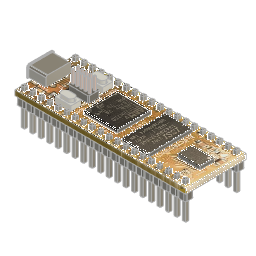
Seed Cover v4 (Autodesk Fusion 360 archive; units mm, degrees)
design "Daisy Board"
Autodesk Fusion 360 part; units mm, degrees
(part 1 of 2)
box "BoxPrimitive1" add length 18.11 width 51.14 height 1.53 placed x (0, -1, 0) y (1, 0, 0) z (0, 0, 1) at (-75.0693, 56.4508, 0) makes body 1
sketch "Sketch3" plane through (0, 0, 1.53) normal (0, 0, 1) x (-1, 0, 0)
  line L0 (75.0693, -38.3408) -> (23.9293, -38.3408)
  line L1 (23.9293, -38.3408) -> (23.9293, -56.4508)
  line L2 (23.9293, -56.4508) -> (75.0693, -56.4508)
  line L3 (75.0693, -56.4508) -> (75.0693, -38.3408)
  line L4 (23.9293, -47.3958) -> (37.4493, -47.3958) construction
  line L5 (37.4493, -56.4508) -> (37.4493, -38.3408) construction
  line L6 (37.4493, -47.3958) -> (45.4493, -47.3958) construction
  line L7 (45.4493, -56.4508) -> (45.4493, -38.3408) construction
  line L8 (45.4493, -47.3958) -> (48.3593, -47.3958) construction
  line L9 (48.3593, -56.4508) -> (48.3593, -38.3408) construction
  line L10 (48.3593, -47.3958) -> (58.3893, -47.3958) construction
  line L11 (58.3893, -56.4508) -> (58.3893, -38.3408) construction
  line L12 (58.3893, -47.3958) -> (60.3893, -47.3958) construction
  line L13 (60.3893, -56.4508) -> (60.3893, -38.3408) construction
  line L14 (60.3893, -47.3958) -> (66.5893, -47.3958) construction
  line L15 (66.5893, -56.4508) -> (66.5893, -38.3408) construction
  line L16 (66.5893, -47.3958) -> (71.0293, -47.3958) construction
  line L17 (71.0293, -56.4508) -> (71.0293, -38.3408) construction
  line L18 (71.0293, -47.3958) -> (76.5893, -47.3958) construction
  line L19 (76.5893, -56.4508) -> (76.5893, -38.3408) construction
  line L20 (23.9293, -47.3958) -> (26.5293, -47.3958) construction
  line L21 (26.5293, -56.4508) -> (26.5293, -38.3408) construction
  line L22 (26.5293, -47.3958) -> (33.1493, -47.3958) construction
  line L23 (33.1493, -56.4508) -> (33.1493, -38.3408) construction
  line L24 (33.1493, -47.3958) -> (33.1493, -49.5458) construction
  line L25 (33.1493, -47.3958) -> (33.1493, -45.2458) construction
  line L26 (33.1493, -49.5458) -> (26.5293, -49.5458)
  line L27 (26.5293, -49.5458) -> (26.5293, -45.2458)
  line L28 (26.5293, -45.2458) -> (33.1493, -45.2458)
  line L29 (33.1493, -45.2458) -> (33.1493, -49.5458)
  line L30 (37.4493, -47.3958) -> (37.4493, -53.8958) construction
  line L31 (37.4493, -47.3958) -> (37.4493, -40.8958) construction
  line L32 (37.4493, -53.8958) -> (45.4493, -53.8958)
  line L33 (45.4493, -53.8958) -> (45.4493, -40.8958)
  line L34 (45.4493, -40.8958) -> (37.4493, -40.8958)
  line L35 (37.4493, -40.8958) -> (37.4493, -53.8958)
  line L36 (48.3593, -47.3958) -> (48.3593, -52.4158) construction
  line L37 (48.3593, -47.3958) -> (48.3593, -42.3758) construction
  line L38 (48.3593, -52.4158) -> (58.3893, -52.4158)
  line L39 (58.3893, -52.4158) -> (58.3893, -42.3758)
  line L40 (58.3893, -42.3758) -> (48.3593, -42.3758)
  line L41 (48.3593, -42.3758) -> (48.3593, -52.4158)
  line L42 (60.3893, -47.3958) -> (60.3893, -49.0758) construction
  line L43 (60.3893, -47.3958) -> (60.3893, -45.7158) construction
  line L44 (60.3893, -45.7158) -> (66.5893, -45.7158)
  line L45 (66.5893, -45.7158) -> (66.5893, -49.0758)
  line L46 (66.5893, -49.0758) -> (60.3893, -49.0758)
  line L47 (60.3893, -49.0758) -> (60.3893, -45.7158)
  line L48 (71.0293, -47.3958) -> (71.0293, -51.1708) construction
  line L49 (71.0293, -47.3958) -> (71.0293, -43.6208) construction
  line L50 (71.0293, -51.1708) -> (76.5893, -51.1708)
  line L51 (76.5893, -51.1708) -> (76.5893, -43.6208)
  line L52 (76.5893, -43.6208) -> (71.0293, -43.6208)
  line L53 (71.0293, -43.6208) -> (71.0293, -51.1708)
  line L54 (66.5893, -49.0758) -> (66.5893, -50.5758) construction
  line L55 (66.5893, -45.7158) -> (66.5893, -44.2158) construction
  line L56 (65.9033, -38.3408) -> (65.9033, -56.4508) construction
  line L57 (61.0338, -38.3408) -> (61.0338, -56.4508) construction
  line L58 (65.9033, -50.5758) -> (61.0338, -50.5758)
  line L59 (61.0338, -50.5758) -> (61.0338, -53.7158)
  line L60 (61.0338, -53.7158) -> (65.9033, -53.7158)
  line L61 (65.9033, -53.7158) -> (65.9033, -50.5758)
  line L62 (65.9033, -44.2158) -> (61.0338, -44.2158)
  line L63 (61.0338, -44.2158) -> (61.0338, -41.0758)
  line L64 (61.0338, -41.0758) -> (65.9033, -41.0758)
  line L65 (65.9033, -41.0758) -> (65.9033, -44.2158)
  line L66 (64.4033, -51.0758) -> (62.5338, -51.0758)
  line L67 (61.5338, -52.0758) -> (61.5338, -52.2158)
  line L68 (62.5338, -53.2158) -> (64.4033, -53.2158)
  line L69 (65.4033, -52.2158) -> (65.4033, -52.0758)
  line L70 (62.5338, -41.5758) -> (64.4033, -41.5758)
  line L71 (65.4033, -42.5758) -> (65.4033, -42.7158)
  line L72 (64.4033, -43.7158) -> (62.5338, -43.7158)
  line L73 (61.5338, -42.7158) -> (61.5338, -42.5758)
  arc A0 (64.4033, -53.2158) -> (65.4033, -52.2158) centre (64.4033, -52.2158) ccw
  arc A1 (61.5338, -52.2158) -> (62.5338, -53.2158) centre (62.5338, -52.2158) ccw
  arc A2 (62.5338, -51.0758) -> (61.5338, -52.0758) centre (62.5338, -52.0758) ccw
  arc A3 (65.4033, -52.0758) -> (64.4033, -51.0758) centre (64.4033, -52.0758) ccw
  arc A4 (64.4033, -43.7158) -> (65.4033, -42.7158) centre (64.4033, -42.7158) ccw
  arc A5 (61.5338, -42.7158) -> (62.5338, -43.7158) centre (62.5338, -42.7158) ccw
  arc A6 (62.5338, -41.5758) -> (61.5338, -42.5758) centre (62.5338, -42.5758) ccw
  arc A7 (65.4033, -42.5758) -> (64.4033, -41.5758) centre (64.4033, -42.5758) ccw
  dimension "d7" = 13.52
  dimension "d8" = 8
  dimension "d9" = 2.91
  dimension "d10" = 10.03
  dimension "d11" = 2
  dimension "d12" = 6.2
  dimension "d13" = 4.44
  dimension "d14" = 5.56
  dimension "d15" = 2.6
  dimension "d16" = 6.62
  dimension "d17" = 2.15
  dimension "d18" = 2.15
  dimension "d19" = 6.5
  dimension "d20" = 6.5
  dimension "d21" = 5.02
  dimension "d22" = 5.02
  dimension "d23" = 1.68
  dimension "d24" = 1.68
  dimension "d25" = 3.775
  dimension "d26" = 3.775
  dimension "d49" = 1.5
  dimension "d50" = 1.5
  dimension "d51" = 3.14
  dimension "d52" = 3.14
  dimension "d55" = 1
  constraint midpoint L1 L4.start
  constraint perpendicular L1 L4
  constraint coincident L2 L5.start
  constraint coincident L0 L5.end
  constraint perpendicular L0 L5
  constraint perpendicular L5 L6
  constraint coincident L2 L7.start
  constraint coincident L0 L7.end
  constraint perpendicular L0 L7
  constraint perpendicular L7 L8
  constraint coincident L2 L9.start
  constraint coincident L0 L9.end
  constraint perpendicular L0 L9
  constraint perpendicular L9 L10
  constraint coincident L2 L11.start
  constraint coincident L0 L11.end
  constraint perpendicular L0 L11
  constraint perpendicular L11 L12
  constraint coincident L2 L13.start
  constraint coincident L0 L13.end
  constraint perpendicular L0 L13
  constraint perpendicular L13 L14
  constraint coincident L2 L15.start
  constraint coincident L0 L15.end
  constraint perpendicular L0 L15
  constraint perpendicular L15 L16
  constraint coincident L2 L17.start
  constraint coincident L0 L17.end
  constraint perpendicular L0 L17
  constraint perpendicular L3 L18
  constraint perpendicular L0 L19
  constraint perpendicular L1 L20
  constraint coincident L2 L21.start
  constraint coincident L0 L21.end
  constraint perpendicular L0 L21
  constraint perpendicular L21 L22
  constraint coincident L2 L23.start
  constraint coincident L0 L23.end
  constraint perpendicular L0 L23
  constraint perpendicular L4 L24
  constraint perpendicular L4 L25
  constraint horizontal L26
  constraint vertical L27
  constraint horizontal L28
  constraint vertical L29
  constraint coincident L21 L27.end
  constraint perpendicular L6 L30
  constraint perpendicular L6 L31
  constraint horizontal L32
  constraint vertical L33
  constraint horizontal L34
  constraint vertical L35
  constraint coincident L7 L33.end
  constraint perpendicular L10 L36
  constraint perpendicular L10 L37
  constraint horizontal L38
  constraint vertical L39
  constraint horizontal L40
  constraint vertical L41
  constraint coincident L11 L39.end
  constraint perpendicular L14 L42
  constraint perpendicular L14 L43
  constraint horizontal L44
  constraint vertical L45
  constraint horizontal L46
  constraint vertical L47
  constraint coincident L15 L45.end
  constraint perpendicular L18 L48
  constraint perpendicular L16 L49
  constraint horizontal L50
  constraint vertical L51
  constraint horizontal L52
  constraint vertical L53
  constraint coincident L19 L51.end
  constraint perpendicular L46 L54
  constraint perpendicular L44 L55
  constraint coincident L0 L56.start
  constraint coincident L2 L56.end
  constraint perpendicular L2 L56
  constraint coincident L0 L57.start
  constraint perpendicular L46 L57
  constraint horizontal L58
  constraint vertical L59
  constraint horizontal L60
  constraint vertical L61
  constraint coincident L56 L58.start
  constraint horizontal L62
  constraint vertical L63
  constraint horizontal L64
  constraint vertical L65
  constraint coincident L56 L62.start
  constraint parallel L58 L66
  constraint parallel L59 L67
  constraint parallel L60 L68
  constraint parallel L61 L69
  constraint tangent L68 A0
  constraint tangent L69 A0
  constraint tangent L67 A1
  constraint tangent L68 A1
  constraint equal A0 A1
  constraint tangent L66 A2
  constraint tangent L67 A2
  constraint equal A0 A2
  constraint tangent L66 A3
  constraint tangent L69 A3
  constraint equal A0 A3
  constraint parallel L64 L70
  constraint parallel L65 L71
  constraint parallel L62 L72
  constraint parallel L63 L73
  constraint tangent L71 A4
  constraint tangent L72 A4
  constraint equal A0 A4
  constraint tangent L72 A5
  constraint tangent L73 A5
  constraint equal A0 A5
  constraint tangent L70 A6
  constraint tangent L73 A6
  constraint equal A0 A6
  constraint tangent L70 A7
  constraint tangent L71 A7
  constraint equal A0 A7
  measures "d7" distance of L4.start L4.end
  measures "d8" distance of L4.end L6.end
  measures "d9" distance of L6.end L8.end
  measures "d10" distance of L8.end L10.end
  measures "d11" distance of L10.end L12.end
  measures "d12" distance of L12.end L14.end
  measures "d13" distance of L14.end L16.end
  measures "d14" distance of L16.end L18.end
  measures "d15" distance of L4.start L20.end
  measures "d16" distance of L20.end L22.end
  measures "d17" distance of L22.end L24.end
  measures "d18" distance of L22.end L25.end
  measures "d19" distance of L4.end L30.end
  measures "d20" distance of L4.end L31.end
  measures "d21" distance of L8.end L36.end
  measures "d22" distance of L8.end L37.end
  measures "d23" distance of L12.end L42.end
  measures "d24" distance of L12.end L43.end
  measures "d25" distance of L16.end L48.end
  measures "d26" distance of L16.end L49.end
  measures "d49" distance of L45.end L54.end
  measures "d50" distance of L44.end L55.end
  measures "d51" distance of L58.start L60.end
  measures "d52" distance of L62.start L64.end
  measures "d55" radius of A0
extrude "Extrude1" add sketch "Sketch3" along normal blind 1 separate body contours L26 L27 L28 L29 makes body 2
extrude "Extrude2" add sketch "Sketch3" along normal blind 1 separate body contours L32 L33 L34 L35 makes body 3
extrude "Extrude3" add sketch "Sketch3" along normal blind 1 separate body contours L38 L39 L40 L41 makes body 4
extrude "Extrude4" add sketch "Sketch3" along normal blind 2 separate body contours L44 L45 L46 L47 makes body 5
extrude "Extrude5" add sketch "Sketch3" along normal blind 3 separate body contours L3 L50 L51 L52 | L3 L50 L52 L53 makes body 6
fillet "Fillet1" radius 0.5 2 edges at (-73.8093, 51.1708, 4.53) (-73.8093, 43.6208, 4.53) on bodies 6
fillet "Fillet2" radius 0.25 tangency weight 0.80688 4 edges at (-66.5893, 45.7158, 2.53) (-66.5893, 49.0758, 2.53) (-60.3893, 49.0758, 2.53) (-60.3893, 45.7158, 2.53) on bodies 5
sketch "Sketch4" plane through (0, 0, 3.53) normal (0, 0, 1) x (-1, 0, 0)
  spline S0 degree 3 poles (60.3893, -45.9658) (60.3893, -45.9427) (60.3942, -45.9181) (60.4159, -45.8622) (60.435, -45.8319) (60.4862, -45.776) (60.5184, -45.7522) (60.5671, -45.7296) (60.5826, -45.7241) (60.6118, -45.7175) (60.6256, -45.7158) (60.6393, -45.7158) knots 0 0 0 0 0.006926 0.006926 0.015648 0.015648 0.025212 0.025212 0.029372 0.029372 0.032888 0.032888 0.032888 0.032888
  line L0 (60.3893, -45.9658) -> (60.3893, -48.8258)
  spline S1 degree 3 poles (60.6393, -49.0758) (60.6162, -49.0758) (60.5917, -49.0709) (60.5358, -49.0492) (60.5055, -49.03) (60.4495, -48.9788) (60.4257, -48.9467) (60.4032, -48.898) (60.3977, -48.8825) (60.391, -48.8532) (60.3893, -48.8395) (60.3893, -48.8258) knots 0 0 0 0 0.006926 0.006926 0.015648 0.015648 0.025212 0.025212 0.029372 0.029372 0.032888 0.032888 0.032888 0.032888
  line L1 (60.6393, -49.0758) -> (66.3393, -49.0758)
  spline S2 degree 3 poles (66.5893, -48.8258) (66.5893, -48.8488) (66.5844, -48.8734) (66.5627, -48.9293) (66.5436, -48.9596) (66.4924, -49.0156) (66.4602, -49.0394) (66.4115, -49.0619) (66.396, -49.0674) (66.3668, -49.074) (66.353, -49.0758) (66.3393, -49.0758) knots 0 0 0 0 0.006926 0.006926 0.015648 0.015648 0.025212 0.025212 0.029372 0.029372 0.032888 0.032888 0.032888 0.032888
  line L2 (66.5893, -48.8258) -> (66.5893, -45.9658)
  spline S3 degree 3 poles (66.3393, -45.7158) (66.3624, -45.7158) (66.387, -45.7207) (66.4429, -45.7423) (66.4732, -45.7615) (66.5291, -45.8127) (66.5529, -45.8448) (66.5754, -45.8936) (66.5809, -45.9091) (66.5876, -45.9383) (66.5893, -45.952) (66.5893, -45.9658) knots 0 0 0 0 0.006926 0.006926 0.015648 0.015648 0.025212 0.025212 0.029372 0.029372 0.032888 0.032888 0.032888 0.032888
  line L3 (66.3393, -45.7158) -> (60.6393, -45.7158)
  line L4 (65.7564, -47.944) -> (66.2564, -47.944)
  line L5 (66.2564, -47.944) -> (66.2564, -48.444)
  line L6 (66.2564, -48.444) -> (65.7564, -48.444)
  line L7 (65.7564, -48.444) -> (65.7564, -47.944)
  line L8 (65.7564, -47.944) -> (66.2564, -48.444) construction
  line L9 (66.2564, -47.944) -> (65.7564, -48.444) construction
  line L10 (65.0064, -48.444) -> (64.5064, -48.444)
  line L11 (64.5064, -47.944) -> (65.0064, -47.944)
  line L12 (64.5064, -48.444) -> (64.5064, -47.944)
  line L13 (65.0064, -47.944) -> (65.0064, -48.444)
  line L14 (63.7564, -48.444) -> (63.2564, -48.444)
  line L15 (63.2564, -47.944) -> (63.7564, -47.944)
  line L16 (63.2564, -48.444) -> (63.2564, -47.944)
  line L17 (63.7564, -47.944) -> (63.7564, -48.444)
  line L18 (62.5064, -48.444) -> (62.0064, -48.444)
  line L19 (62.0064, -47.944) -> (62.5064, -47.944)
  line L20 (62.0064, -48.444) -> (62.0064, -47.944)
  line L21 (62.5064, -47.944) -> (62.5064, -48.444)
  line L22 (61.2564, -48.444) -> (60.7564, -48.444)
  line L23 (60.7564, -47.944) -> (61.2564, -47.944)
  line L24 (60.7564, -48.444) -> (60.7564, -47.944)
  line L25 (61.2564, -47.944) -> (61.2564, -48.444)
  line L26 (66.2564, -46.944) -> (65.7564, -46.944)
  line L27 (65.7564, -46.444) -> (66.2564, -46.444)
  line L28 (65.7564, -46.944) -> (65.7564, -46.444)
  line L29 (66.2564, -46.444) -> (66.2564, -46.944)
  line L30 (65.0064, -46.944) -> (64.5064, -46.944)
  line L31 (64.5064, -46.444) -> (65.0064, -46.444)
  line L32 (64.5064, -46.944) -> (64.5064, -46.444)
  line L33 (65.0064, -46.444) -> (65.0064, -46.944)
  line L34 (63.7564, -46.944) -> (63.2564, -46.944)
  line L35 (63.2564, -46.444) -> (63.7564, -46.444)
  line L36 (63.2564, -46.944) -> (63.2564, -46.444)
  line L37 (63.7564, -46.444) -> (63.7564, -46.944)
  line L38 (62.5064, -46.944) -> (62.0064, -46.944)
  line L39 (62.0064, -46.444) -> (62.5064, -46.444)
  line L40 (62.0064, -46.944) -> (62.0064, -46.444)
  line L41 (62.5064, -46.444) -> (62.5064, -46.944)
  line L42 (61.2564, -46.944) -> (60.7564, -46.944)
  line L43 (60.7564, -46.444) -> (61.2564, -46.444)
  line L44 (60.7564, -46.944) -> (60.7564, -46.444)
  line L45 (61.2564, -46.444) -> (61.2564, -46.944)
  point P0 (66.0064, -48.194)
  dimension "d41" = 0.5
  dimension "d42" = 0.5
  dimension "d45" = -5
  dimension "d46" = 1.5
  constraint horizontal L4
  constraint perpendicular L4 L5
  constraint parallel L4 L6
  constraint parallel L5 L7
  constraint coincident L8 P0
  constraint coincident L9 P0
  measures "d41" distance of L5.end L6.end
  measures "d42" distance of L4.end L5.end
extrude "Extrude6" add sketch "Sketch4" along normal blind 4 separate body contours L4 L5 L6 L7 | L10 L11 L12 L13 | L14 L15 L16 L17 | L18 L19 L20 L21 | L22 L23 L24 L25 | L26 L27 L28 L29 | L30 L31 L32 L33 | L34 L35 L36 L37 | L38 L39 L40 L41 | L42 L43 L44 L45 makes body 7 at (-63.5898, 46.944, 4.8633) makes body 8 at (-62.3398, 48.444, 4.8633) makes body 9 at (-64.5064, 48.2774, 4.8633) makes body 10 at (-61.0898, 48.444, 4.8633) makes body 11 at (-64.5064, 46.7774, 4.8633) makes body 12 at (-62.3398, 46.944, 4.8633) makes body 13 at (-63.5898, 48.444, 4.8633) makes body 14 at (-66.2564, 48.1107, 4.8633) makes body 15 at (-61.0898, 46.944, 4.8633) makes body 16 at (-65.7564, 46.7774, 4.8633)
extrude "Extrude7" add sketch "Sketch3" along normal blind 1.5 separate body contours L58 L59 L60 L61 | L62 L63 L64 L65 makes body 17 at (-63.7801, 44.0491, 1.53) makes body 18 at (-63.157, 53.5491, 1.53)
extrude "Extrude8" add sketch "Sketch3" along normal blind 2.5 separate body contours L66 L67 L68 L69 A0 A1 A2 A3 | L70 L71 L72 L73 A4 A5 A6 A7 makes body 19 at (-63.7801, 52.5024, 1.53) makes body 20 at (-63.157, 43.0024, 1.53)
shell "Shell1" thickness 0.3 removed faces 1 at (-76.5893, 48.4874, 2.53) on bodies 6
sketch "Sketch5" plane through (0, 0, 0) normal (0, 0, -1) x (1, 0, 0)
  line L0 (-23.9293, -38.3408) -> (-75.0693, -38.3408)
  line L1 (-75.0693, -38.3408) -> (-75.0693, -56.4508)
  line L2 (-75.0693, -56.4508) -> (-23.9293, -56.4508)
  line L3 (-23.9293, -56.4508) -> (-23.9293, -38.3408)
  line L4 (-74.3757, -41.0103) -> (-72.8757, -41.0103)
  line L5 (-72.3757, -40.5103) -> (-72.3757, -39.0103)
  line L6 (-72.8757, -38.5103) -> (-74.3757, -38.5103)
  line L7 (-74.8757, -39.0103) -> (-74.8757, -40.5103)
  line L8 (-74.1023, -40.2369) -> (-73.1491, -40.2369)
  line L9 (-73.1491, -40.2369) -> (-73.1491, -39.2838)
  line L10 (-73.1491, -39.2838) -> (-74.1023, -39.2838)
  line L11 (-74.1023, -39.2838) -> (-74.1023, -40.2369)
  arc A0 (-74.3757, -38.5103) -> (-74.8757, -39.0103) centre (-74.3757, -39.0103) ccw
  arc A1 (-72.3757, -39.0103) -> (-72.8757, -38.5103) centre (-72.8757, -39.0103) ccw
  arc A2 (-72.8757, -41.0103) -> (-72.3757, -40.5103) centre (-72.8757, -40.5103) ccw
  arc A3 (-74.8757, -40.5103) -> (-74.3757, -41.0103) centre (-74.3757, -40.5103) ccw
  arc A4 (-69.8362, -39.0103) -> (-70.3362, -38.5103) centre (-70.3362, -39.0103) ccw
  line L12 (-70.3362, -38.5103) -> (-71.8362, -38.5103)
  line L13 (-72.3362, -39.0103) -> (-72.3362, -40.5103)
  arc A5 (-71.8362, -38.5103) -> (-72.3362, -39.0103) centre (-71.8362, -39.0103) ccw
  line L14 (-71.5628, -39.2838) -> (-71.5628, -40.2369)
  arc A6 (-72.3362, -40.5103) -> (-71.8362, -41.0103) centre (-71.8362, -40.5103) ccw
  line L15 (-70.6097, -39.2838) -> (-71.5628, -39.2838)
  line L16 (-69.8362, -40.5103) -> (-69.8362, -39.0103)
  arc A7 (-70.3362, -41.0103) -> (-69.8362, -40.5103) centre (-70.3362, -40.5103) ccw
  line L17 (-70.6097, -40.2369) -> (-70.6097, -39.2838)
  line L18 (-71.5628, -40.2369) -> (-70.6097, -40.2369)
  line L19 (-71.8362, -41.0103) -> (-70.3362, -41.0103)
  arc A8 (-67.2968, -39.0103) -> (-67.7968, -38.5103) centre (-67.7968, -39.0103) ccw
  line L20 (-67.7968, -38.5103) -> (-69.2968, -38.5103)
  line L21 (-69.7968, -39.0103) -> (-69.7968, -40.5103)
  arc A9 (-69.2968, -38.5103) -> (-69.7968, -39.0103) centre (-69.2968, -39.0103) ccw
  line L22 (-69.0233, -39.2838) -> (-69.0233, -40.2369)
  arc A10 (-69.7968, -40.5103) -> (-69.2968, -41.0103) centre (-69.2968, -40.5103) ccw
  line L23 (-68.0702, -39.2838) -> (-69.0233, -39.2838)
  line L24 (-67.2968, -40.5103) -> (-67.2968, -39.0103)
  arc A11 (-67.7968, -41.0103) -> (-67.2968, -40.5103) centre (-67.7968, -40.5103) ccw
  line L25 (-68.0702, -40.2369) -> (-68.0702, -39.2838)
  line L26 (-69.0233, -40.2369) -> (-68.0702, -40.2369)
  line L27 (-69.2968, -41.0103) -> (-67.7968, -41.0103)
  arc A12 (-64.7573, -39.0103) -> (-65.2573, -38.5103) centre (-65.2573, -39.0103) ccw
  line L28 (-65.2573, -38.5103) -> (-66.7573, -38.5103)
  line L29 (-67.2573, -39.0103) -> (-67.2573, -40.5103)
  arc A13 (-66.7573, -38.5103) -> (-67.2573, -39.0103) centre (-66.7573, -39.0103) ccw
  line L30 (-66.4839, -39.2838) -> (-66.4839, -40.2369)
  arc A14 (-67.2573, -40.5103) -> (-66.7573, -41.0103) centre (-66.7573, -40.5103) ccw
  line L31 (-65.5307, -39.2838) -> (-66.4839, -39.2838)
  line L32 (-64.7573, -40.5103) -> (-64.7573, -39.0103)
  arc A15 (-65.2573, -41.0103) -> (-64.7573, -40.5103) centre (-65.2573, -40.5103) ccw
  line L33 (-65.5307, -40.2369) -> (-65.5307, -39.2838)
  line L34 (-66.4839, -40.2369) -> (-65.5307, -40.2369)
  line L35 (-66.7573, -41.0103) -> (-65.2573, -41.0103)
  arc A16 (-62.2178, -39.0103) -> (-62.7178, -38.5103) centre (-62.7178, -39.0103) ccw
  line L36 (-62.7178, -38.5103) -> (-64.2178, -38.5103)
  line L37 (-64.7178, -39.0103) -> (-64.7178, -40.5103)
  arc A17 (-64.2178, -38.5103) -> (-64.7178, -39.0103) centre (-64.2178, -39.0103) ccw
  line L38 (-63.9444, -39.2838) -> (-63.9444, -40.2369)
  arc A18 (-64.7178, -40.5103) -> (-64.2178, -41.0103) centre (-64.2178, -40.5103) ccw
  line L39 (-62.9912, -39.2838) -> (-63.9444, -39.2838)
  line L40 (-62.2178, -40.5103) -> (-62.2178, -39.0103)
  arc A19 (-62.7178, -41.0103) -> (-62.2178, -40.5103) centre (-62.7178, -40.5103) ccw
  line L41 (-62.9912, -40.2369) -> (-62.9912, -39.2838)
  line L42 (-63.9444, -40.2369) -> (-62.9912, -40.2369)
  line L43 (-64.2178, -41.0103) -> (-62.7178, -41.0103)
  arc A20 (-59.6783, -39.0103) -> (-60.1783, -38.5103) centre (-60.1783, -39.0103) ccw
  line L44 (-60.1783, -38.5103) -> (-61.6783, -38.5103)
  line L45 (-62.1783, -39.0103) -> (-62.1783, -40.5103)
  arc A21 (-61.6783, -38.5103) -> (-62.1783, -39.0103) centre (-61.6783, -39.0103) ccw
  line L46 (-61.4049, -39.2838) -> (-61.4049, -40.2369)
  arc A22 (-62.1783, -40.5103) -> (-61.6783, -41.0103) centre (-61.6783, -40.5103) ccw
  line L47 (-60.4518, -39.2838) -> (-61.4049, -39.2838)
  line L48 (-59.6783, -40.5103) -> (-59.6783, -39.0103)
  arc A23 (-60.1783, -41.0103) -> (-59.6783, -40.5103) centre (-60.1783, -40.5103) ccw
  line L49 (-60.4518, -40.2369) -> (-60.4518, -39.2838)
  line L50 (-61.4049, -40.2369) -> (-60.4518, -40.2369)
  line L51 (-61.6783, -41.0103) -> (-60.1783, -41.0103)
  arc A24 (-57.1389, -39.0103) -> (-57.6389, -38.5103) centre (-57.6389, -39.0103) ccw
  line L52 (-57.6389, -38.5103) -> (-59.1389, -38.5103)
  line L53 (-59.6389, -39.0103) -> (-59.6389, -40.5103)
  arc A25 (-59.1389, -38.5103) -> (-59.6389, -39.0103) centre (-59.1389, -39.0103) ccw
  line L54 (-58.8654, -39.2838) -> (-58.8654, -40.2369)
  arc A26 (-59.6389, -40.5103) -> (-59.1389, -41.0103) centre (-59.1389, -40.5103) ccw
  line L55 (-57.9123, -39.2838) -> (-58.8654, -39.2838)
  line L56 (-57.1389, -40.5103) -> (-57.1389, -39.0103)
  arc A27 (-57.6389, -41.0103) -> (-57.1389, -40.5103) centre (-57.6389, -40.5103) ccw
  line L57 (-57.9123, -40.2369) -> (-57.9123, -39.2838)
  line L58 (-58.8654, -40.2369) -> (-57.9123, -40.2369)
  line L59 (-59.1389, -41.0103) -> (-57.6389, -41.0103)
  arc A28 (-54.5994, -39.0103) -> (-55.0994, -38.5103) centre (-55.0994, -39.0103) ccw
  line L60 (-55.0994, -38.5103) -> (-56.5994, -38.5103)
  line L61 (-57.0994, -39.0103) -> (-57.0994, -40.5103)
  arc A29 (-56.5994, -38.5103) -> (-57.0994, -39.0103) centre (-56.5994, -39.0103) ccw
  line L62 (-56.326, -39.2838) -> (-56.326, -40.2369)
  arc A30 (-57.0994, -40.5103) -> (-56.5994, -41.0103) centre (-56.5994, -40.5103) ccw
  line L63 (-55.3728, -39.2838) -> (-56.326, -39.2838)
  line L64 (-54.5994, -40.5103) -> (-54.5994, -39.0103)
  arc A31 (-55.0994, -41.0103) -> (-54.5994, -40.5103) centre (-55.0994, -40.5103) ccw
  line L65 (-55.3728, -40.2369) -> (-55.3728, -39.2838)
  line L66 (-56.326, -40.2369) -> (-55.3728, -40.2369)
  line L67 (-56.5994, -41.0103) -> (-55.0994, -41.0103)
  arc A32 (-52.0599, -39.0103) -> (-52.5599, -38.5103) centre (-52.5599, -39.0103) ccw
  line L68 (-52.5599, -38.5103) -> (-54.0599, -38.5103)
  line L69 (-54.5599, -39.0103) -> (-54.5599, -40.5103)
  arc A33 (-54.0599, -38.5103) -> (-54.5599, -39.0103) centre (-54.0599, -39.0103) ccw
  line L70 (-53.7865, -39.2838) -> (-53.7865, -40.2369)
  arc A34 (-54.5599, -40.5103) -> (-54.0599, -41.0103) centre (-54.0599, -40.5103) ccw
  line L71 (-52.8333, -39.2838) -> (-53.7865, -39.2838)
  line L72 (-52.0599, -40.5103) -> (-52.0599, -39.0103)
  arc A35 (-52.5599, -41.0103) -> (-52.0599, -40.5103) centre (-52.5599, -40.5103) ccw
  line L73 (-52.8333, -40.2369) -> (-52.8333, -39.2838)
  line L74 (-53.7865, -40.2369) -> (-52.8333, -40.2369)
  line L75 (-54.0599, -41.0103) -> (-52.5599, -41.0103)
  arc A36 (-49.5204, -39.0103) -> (-50.0204, -38.5103) centre (-50.0204, -39.0103) ccw
  line L76 (-50.0204, -38.5103) -> (-51.5204, -38.5103)
  line L77 (-52.0204, -39.0103) -> (-52.0204, -40.5103)
  arc A37 (-51.5204, -38.5103) -> (-52.0204, -39.0103) centre (-51.5204, -39.0103) ccw
  line L78 (-51.247, -39.2838) -> (-51.247, -40.2369)
  arc A38 (-52.0204, -40.5103) -> (-51.5204, -41.0103) centre (-51.5204, -40.5103) ccw
  line L79 (-50.2939, -39.2838) -> (-51.247, -39.2838)
  line L80 (-49.5204, -40.5103) -> (-49.5204, -39.0103)
  arc A39 (-50.0204, -41.0103) -> (-49.5204, -40.5103) centre (-50.0204, -40.5103) ccw
  line L81 (-50.2939, -40.2369) -> (-50.2939, -39.2838)
  line L82 (-51.247, -40.2369) -> (-50.2939, -40.2369)
  line L83 (-51.5204, -41.0103) -> (-50.0204, -41.0103)
  arc A40 (-46.981, -39.0103) -> (-47.481, -38.5103) centre (-47.481, -39.0103) ccw
  line L84 (-47.481, -38.5103) -> (-48.981, -38.5103)
  line L85 (-49.481, -39.0103) -> (-49.481, -40.5103)
  arc A41 (-48.981, -38.5103) -> (-49.481, -39.0103) centre (-48.981, -39.0103) ccw
  line L86 (-48.7076, -39.2838) -> (-48.7076, -40.2369)
  arc A42 (-49.481, -40.5103) -> (-48.981, -41.0103) centre (-48.981, -40.5103) ccw
  line L87 (-47.7544, -39.2838) -> (-48.7076, -39.2838)
  line L88 (-46.981, -40.5103) -> (-46.981, -39.0103)
  arc A43 (-47.481, -41.0103) -> (-46.981, -40.5103) centre (-47.481, -40.5103) ccw
  line L89 (-47.7544, -40.2369) -> (-47.7544, -39.2838)
  line L90 (-48.7076, -40.2369) -> (-47.7544, -40.2369)
  line L91 (-48.981, -41.0103) -> (-47.481, -41.0103)
  arc A44 (-44.4415, -39.0103) -> (-44.9415, -38.5103) centre (-44.9415, -39.0103) ccw
  line L92 (-44.9415, -38.5103) -> (-46.4415, -38.5103)
  line L93 (-46.9415, -39.0103) -> (-46.9415, -40.5103)
  arc A45 (-46.4415, -38.5103) -> (-46.9415, -39.0103) centre (-46.4415, -39.0103) ccw
  line L94 (-46.1681, -39.2838) -> (-46.1681, -40.2369)
  arc A46 (-46.9415, -40.5103) -> (-46.4415, -41.0103) centre (-46.4415, -40.5103) ccw
  line L95 (-45.2149, -39.2838) -> (-46.1681, -39.2838)
  line L96 (-44.4415, -40.5103) -> (-44.4415, -39.0103)
  arc A47 (-44.9415, -41.0103) -> (-44.4415, -40.5103) centre (-44.9415, -40.5103) ccw
  line L97 (-45.2149, -40.2369) -> (-45.2149, -39.2838)
  line L98 (-46.1681, -40.2369) -> (-45.2149, -40.2369)
  line L99 (-46.4415, -41.0103) -> (-44.9415, -41.0103)
  arc A48 (-41.902, -39.0103) -> (-42.402, -38.5103) centre (-42.402, -39.0103) ccw
  line L100 (-42.402, -38.5103) -> (-43.902, -38.5103)
  line L101 (-44.402, -39.0103) -> (-44.402, -40.5103)
  arc A49 (-43.902, -38.5103) -> (-44.402, -39.0103) centre (-43.902, -39.0103) ccw
  line L102 (-43.6286, -39.2838) -> (-43.6286, -40.2369)
  arc A50 (-44.402, -40.5103) -> (-43.902, -41.0103) centre (-43.902, -40.5103) ccw
  line L103 (-42.6755, -39.2838) -> (-43.6286, -39.2838)
  line L104 (-41.902, -40.5103) -> (-41.902, -39.0103)
  arc A51 (-42.402, -41.0103) -> (-41.902, -40.5103) centre (-42.402, -40.5103) ccw
  line L105 (-42.6755, -40.2369) -> (-42.6755, -39.2838)
  line L106 (-43.6286, -40.2369) -> (-42.6755, -40.2369)
  line L107 (-43.902, -41.0103) -> (-42.402, -41.0103)
  arc A52 (-39.3626, -39.0103) -> (-39.8626, -38.5103) centre (-39.8626, -39.0103) ccw
  line L108 (-39.8626, -38.5103) -> (-41.3626, -38.5103)
  line L109 (-41.8626, -39.0103) -> (-41.8626, -40.5103)
  arc A53 (-41.3626, -38.5103) -> (-41.8626, -39.0103) centre (-41.3626, -39.0103) ccw
  line L110 (-41.0891, -39.2838) -> (-41.0891, -40.2369)
  arc A54 (-41.8626, -40.5103) -> (-41.3626, -41.0103) centre (-41.3626, -40.5103) ccw
  line L111 (-40.136, -39.2838) -> (-41.0891, -39.2838)
  line L112 (-39.3626, -40.5103) -> (-39.3626, -39.0103)
  arc A55 (-39.8626, -41.0103) -> (-39.3626, -40.5103) centre (-39.8626, -40.5103) ccw
  line L113 (-40.136, -40.2369) -> (-40.136, -39.2838)
  line L114 (-41.0891, -40.2369) -> (-40.136, -40.2369)
  line L115 (-41.3626, -41.0103) -> (-39.8626, -41.0103)
  arc A56 (-36.8231, -39.0103) -> (-37.3231, -38.5103) centre (-37.3231, -39.0103) ccw
  line L116 (-37.3231, -38.5103) -> (-38.8231, -38.5103)
  line L117 (-39.3231, -39.0103) -> (-39.3231, -40.5103)
  arc A57 (-38.8231, -38.5103) -> (-39.3231, -39.0103) centre (-38.8231, -39.0103) ccw
  line L118 (-38.5497, -39.2838) -> (-38.5497, -40.2369)
  arc A58 (-39.3231, -40.5103) -> (-38.8231, -41.0103) centre (-38.8231, -40.5103) ccw
  line L119 (-37.5965, -39.2838) -> (-38.5497, -39.2838)
  line L120 (-36.8231, -40.5103) -> (-36.8231, -39.0103)
  arc A59 (-37.3231, -41.0103) -> (-36.8231, -40.5103) centre (-37.3231, -40.5103) ccw
  line L121 (-37.5965, -40.2369) -> (-37.5965, -39.2838)
  line L122 (-38.5497, -40.2369) -> (-37.5965, -40.2369)
  line L123 (-38.8231, -41.0103) -> (-37.3231, -41.0103)
  arc A60 (-34.2836, -39.0103) -> (-34.7836, -38.5103) centre (-34.7836, -39.0103) ccw
  line L124 (-34.7836, -38.5103) -> (-36.2836, -38.5103)
  line L125 (-36.7836, -39.0103) -> (-36.7836, -40.5103)
  arc A61 (-36.2836, -38.5103) -> (-36.7836, -39.0103) centre (-36.2836, -39.0103) ccw
  line L126 (-36.0102, -39.2838) -> (-36.0102, -40.2369)
  arc A62 (-36.7836, -40.5103) -> (-36.2836, -41.0103) centre (-36.2836, -40.5103) ccw
  line L127 (-35.057, -39.2838) -> (-36.0102, -39.2838)
  line L128 (-34.2836, -40.5103) -> (-34.2836, -39.0103)
  arc A63 (-34.7836, -41.0103) -> (-34.2836, -40.5103) centre (-34.7836, -40.5103) ccw
  line L129 (-35.057, -40.2369) -> (-35.057, -39.2838)
  line L130 (-36.0102, -40.2369) -> (-35.057, -40.2369)
  line L131 (-36.2836, -41.0103) -> (-34.7836, -41.0103)
  arc A64 (-31.7441, -39.0103) -> (-32.2441, -38.5103) centre (-32.2441, -39.0103) ccw
  line L132 (-32.2441, -38.5103) -> (-33.7441, -38.5103)
  line L133 (-34.2441, -39.0103) -> (-34.2441, -40.5103)
  arc A65 (-33.7441, -38.5103) -> (-34.2441, -39.0103) centre (-33.7441, -39.0103) ccw
  line L134 (-33.4707, -39.2838) -> (-33.4707, -40.2369)
  arc A66 (-34.2441, -40.5103) -> (-33.7441, -41.0103) centre (-33.7441, -40.5103) ccw
  line L135 (-32.5176, -39.2838) -> (-33.4707, -39.2838)
  line L136 (-31.7441, -40.5103) -> (-31.7441, -39.0103)
  arc A67 (-32.2441, -41.0103) -> (-31.7441, -40.5103) centre (-32.2441, -40.5103) ccw
  line L137 (-32.5176, -40.2369) -> (-32.5176, -39.2838)
  line L138 (-33.4707, -40.2369) -> (-32.5176, -40.2369)
  line L139 (-33.7441, -41.0103) -> (-32.2441, -41.0103)
  arc A68 (-29.2047, -39.0103) -> (-29.7047, -38.5103) centre (-29.7047, -39.0103) ccw
  line L140 (-29.7047, -38.5103) -> (-31.2047, -38.5103)
  line L141 (-31.7047, -39.0103) -> (-31.7047, -40.5103)
  arc A69 (-31.2047, -38.5103) -> (-31.7047, -39.0103) centre (-31.2047, -39.0103) ccw
  line L142 (-30.9312, -39.2838) -> (-30.9312, -40.2369)
  arc A70 (-31.7047, -40.5103) -> (-31.2047, -41.0103) centre (-31.2047, -40.5103) ccw
  line L143 (-29.9781, -39.2838) -> (-30.9312, -39.2838)
  line L144 (-29.2047, -40.5103) -> (-29.2047, -39.0103)
  arc A71 (-29.7047, -41.0103) -> (-29.2047, -40.5103) centre (-29.7047, -40.5103) ccw
  line L145 (-29.9781, -40.2369) -> (-29.9781, -39.2838)
  line L146 (-30.9312, -40.2369) -> (-29.9781, -40.2369)
  line L147 (-31.2047, -41.0103) -> (-29.7047, -41.0103)
  arc A72 (-26.6652, -39.0103) -> (-27.1652, -38.5103) centre (-27.1652, -39.0103) ccw
  line L148 (-27.1652, -38.5103) -> (-28.6652, -38.5103)
  line L149 (-29.1652, -39.0103) -> (-29.1652, -40.5103)
  arc A73 (-28.6652, -38.5103) -> (-29.1652, -39.0103) centre (-28.6652, -39.0103) ccw
  line L150 (-28.3918, -39.2838) -> (-28.3918, -40.2369)
  arc A74 (-29.1652, -40.5103) -> (-28.6652, -41.0103) centre (-28.6652, -40.5103) ccw
  line L151 (-27.4386, -39.2838) -> (-28.3918, -39.2838)
  line L152 (-26.6652, -40.5103) -> (-26.6652, -39.0103)
  arc A75 (-27.1652, -41.0103) -> (-26.6652, -40.5103) centre (-27.1652, -40.5103) ccw
  line L153 (-27.4386, -40.2369) -> (-27.4386, -39.2838)
  line L154 (-28.3918, -40.2369) -> (-27.4386, -40.2369)
  line L155 (-28.6652, -41.0103) -> (-27.1652, -41.0103)
  arc A76 (-24.1257, -39.0103) -> (-24.6257, -38.5103) centre (-24.6257, -39.0103) ccw
  line L156 (-24.6257, -38.5103) -> (-26.1257, -38.5103)
  line L157 (-26.6257, -39.0103) -> (-26.6257, -40.5103)
  arc A77 (-26.1257, -38.5103) -> (-26.6257, -39.0103) centre (-26.1257, -39.0103) ccw
  line L158 (-25.8523, -39.2838) -> (-25.8523, -40.2369)
  arc A78 (-26.6257, -40.5103) -> (-26.1257, -41.0103) centre (-26.1257, -40.5103) ccw
  line L159 (-24.8991, -39.2838) -> (-25.8523, -39.2838)
  line L160 (-24.1257, -40.5103) -> (-24.1257, -39.0103)
  arc A79 (-24.6257, -41.0103) -> (-24.1257, -40.5103) centre (-24.6257, -40.5103) ccw
  line L161 (-24.8991, -40.2369) -> (-24.8991, -39.2838)
  line L162 (-25.8523, -40.2369) -> (-24.8991, -40.2369)
  line L163 (-26.1257, -41.0103) -> (-24.6257, -41.0103)
  arc A80 (-72.3757, -54.3103) -> (-72.8757, -53.8103) centre (-72.8757, -54.3103) ccw
  line L164 (-72.8757, -53.8103) -> (-74.3757, -53.8103)
  line L165 (-74.8757, -54.3103) -> (-74.8757, -55.8103)
  arc A81 (-74.3757, -53.8103) -> (-74.8757, -54.3103) centre (-74.3757, -54.3103) ccw
  line L166 (-74.1023, -54.5838) -> (-74.1023, -55.5369)
  arc A82 (-74.8757, -55.8103) -> (-74.3757, -56.3103) centre (-74.3757, -55.8103) ccw
  line L167 (-73.1491, -54.5838) -> (-74.1023, -54.5838)
  line L168 (-72.3757, -55.8103) -> (-72.3757, -54.3103)
  arc A83 (-72.8757, -56.3103) -> (-72.3757, -55.8103) centre (-72.8757, -55.8103) ccw
  line L169 (-73.1491, -55.5369) -> (-73.1491, -54.5838)
  line L170 (-74.1023, -55.5369) -> (-73.1491, -55.5369)
  line L171 (-74.3757, -56.3103) -> (-72.8757, -56.3103)
  arc A84 (-69.8362, -54.3103) -> (-70.3362, -53.8103) centre (-70.3362, -54.3103) ccw
  line L172 (-70.3362, -53.8103) -> (-71.8362, -53.8103)
  line L173 (-72.3362, -54.3103) -> (-72.3362, -55.8103)
  arc A85 (-71.8362, -53.8103) -> (-72.3362, -54.3103) centre (-71.8362, -54.3103) ccw
  line L174 (-71.5628, -54.5838) -> (-71.5628, -55.5369)
  arc A86 (-72.3362, -55.8103) -> (-71.8362, -56.3103) centre (-71.8362, -55.8103) ccw
  line L175 (-70.6097, -54.5838) -> (-71.5628, -54.5838)
  line L176 (-69.8362, -55.8103) -> (-69.8362, -54.3103)
  arc A87 (-70.3362, -56.3103) -> (-69.8362, -55.8103) centre (-70.3362, -55.8103) ccw
  line L177 (-70.6097, -55.5369) -> (-70.6097, -54.5838)
  line L178 (-71.5628, -55.5369) -> (-70.6097, -55.5369)
  line L179 (-71.8362, -56.3103) -> (-70.3362, -56.3103)
  arc A88 (-67.2968, -54.3103) -> (-67.7968, -53.8103) centre (-67.7968, -54.3103) ccw
  line L180 (-67.7968, -53.8103) -> (-69.2968, -53.8103)
  line L181 (-69.7968, -54.3103) -> (-69.7968, -55.8103)
  arc A89 (-69.2968, -53.8103) -> (-69.7968, -54.3103) centre (-69.2968, -54.3103) ccw
  line L182 (-69.0233, -54.5838) -> (-69.0233, -55.5369)
  arc A90 (-69.7968, -55.8103) -> (-69.2968, -56.3103) centre (-69.2968, -55.8103) ccw
  line L183 (-68.0702, -54.5838) -> (-69.0233, -54.5838)
  line L184 (-67.2968, -55.8103) -> (-67.2968, -54.3103)
  arc A91 (-67.7968, -56.3103) -> (-67.2968, -55.8103) centre (-67.7968, -55.8103) ccw
  line L185 (-68.0702, -55.5369) -> (-68.0702, -54.5838)
  line L186 (-69.0233, -55.5369) -> (-68.0702, -55.5369)
  line L187 (-69.2968, -56.3103) -> (-67.7968, -56.3103)
  arc A92 (-64.7573, -54.3103) -> (-65.2573, -53.8103) centre (-65.2573, -54.3103) ccw
  line L188 (-65.2573, -53.8103) -> (-66.7573, -53.8103)
  line L189 (-67.2573, -54.3103) -> (-67.2573, -55.8103)
  arc A93 (-66.7573, -53.8103) -> (-67.2573, -54.3103) centre (-66.7573, -54.3103) ccw
  line L190 (-66.4839, -54.5838) -> (-66.4839, -55.5369)
  arc A94 (-67.2573, -55.8103) -> (-66.7573, -56.3103) centre (-66.7573, -55.8103) ccw
  line L191 (-65.5307, -54.5838) -> (-66.4839, -54.5838)
  line L192 (-64.7573, -55.8103) -> (-64.7573, -54.3103)
  arc A95 (-65.2573, -56.3103) -> (-64.7573, -55.8103) centre (-65.2573, -55.8103) ccw
  line L193 (-65.5307, -55.5369) -> (-65.5307, -54.5838)
  line L194 (-66.4839, -55.5369) -> (-65.5307, -55.5369)
  line L195 (-66.7573, -56.3103) -> (-65.2573, -56.3103)
  arc A96 (-62.2178, -54.3103) -> (-62.7178, -53.8103) centre (-62.7178, -54.3103) ccw
  line L196 (-62.7178, -53.8103) -> (-64.2178, -53.8103)
  line L197 (-64.7178, -54.3103) -> (-64.7178, -55.8103)
  arc A97 (-64.2178, -53.8103) -> (-64.7178, -54.3103) centre (-64.2178, -54.3103) ccw
  line L198 (-63.9444, -54.5838) -> (-63.9444, -55.5369)
  arc A98 (-64.7178, -55.8103) -> (-64.2178, -56.3103) centre (-64.2178, -55.8103) ccw
  line L199 (-62.9912, -54.5838) -> (-63.9444, -54.5838)
  line L200 (-62.2178, -55.8103) -> (-62.2178, -54.3103)
  arc A99 (-62.7178, -56.3103) -> (-62.2178, -55.8103) centre (-62.7178, -55.8103) ccw
  line L201 (-62.9912, -55.5369) -> (-62.9912, -54.5838)
  line L202 (-63.9444, -55.5369) -> (-62.9912, -55.5369)
  line L203 (-64.2178, -56.3103) -> (-62.7178, -56.3103)
  arc A100 (-59.6783, -54.3103) -> (-60.1783, -53.8103) centre (-60.1783, -54.3103) ccw
  line L204 (-60.1783, -53.8103) -> (-61.6783, -53.8103)
  line L205 (-62.1783, -54.3103) -> (-62.1783, -55.8103)
  arc A101 (-61.6783, -53.8103) -> (-62.1783, -54.3103) centre (-61.6783, -54.3103) ccw
  line L206 (-61.4049, -54.5838) -> (-61.4049, -55.5369)
  arc A102 (-62.1783, -55.8103) -> (-61.6783, -56.3103) centre (-61.6783, -55.8103) ccw
  line L207 (-60.4518, -54.5838) -> (-61.4049, -54.5838)
  line L208 (-59.6783, -55.8103) -> (-59.6783, -54.3103)
  arc A103 (-60.1783, -56.3103) -> (-59.6783, -55.8103) centre (-60.1783, -55.8103) ccw
  line L209 (-60.4518, -55.5369) -> (-60.4518, -54.5838)
  line L210 (-61.4049, -55.5369) -> (-60.4518, -55.5369)
  line L211 (-61.6783, -56.3103) -> (-60.1783, -56.3103)
  arc A104 (-57.1389, -54.3103) -> (-57.6389, -53.8103) centre (-57.6389, -54.3103) ccw
  line L212 (-57.6389, -53.8103) -> (-59.1389, -53.8103)
  line L213 (-59.6389, -54.3103) -> (-59.6389, -55.8103)
  arc A105 (-59.1389, -53.8103) -> (-59.6389, -54.3103) centre (-59.1389, -54.3103) ccw
  line L214 (-58.8654, -54.5838) -> (-58.8654, -55.5369)
  arc A106 (-59.6389, -55.8103) -> (-59.1389, -56.3103) centre (-59.1389, -55.8103) ccw
  line L215 (-57.9123, -54.5838) -> (-58.8654, -54.5838)
  line L216 (-57.1389, -55.8103) -> (-57.1389, -54.3103)
  arc A107 (-57.6389, -56.3103) -> (-57.1389, -55.8103) centre (-57.6389, -55.8103) ccw
  line L217 (-57.9123, -55.5369) -> (-57.9123, -54.5838)
  line L218 (-58.8654, -55.5369) -> (-57.9123, -55.5369)
  line L219 (-59.1389, -56.3103) -> (-57.6389, -56.3103)
  arc A108 (-54.5994, -54.3103) -> (-55.0994, -53.8103) centre (-55.0994, -54.3103) ccw
  line L220 (-55.0994, -53.8103) -> (-56.5994, -53.8103)
  line L221 (-57.0994, -54.3103) -> (-57.0994, -55.8103)
  arc A109 (-56.5994, -53.8103) -> (-57.0994, -54.3103) centre (-56.5994, -54.3103) ccw
  line L222 (-56.326, -54.5838) -> (-56.326, -55.5369)
  arc A110 (-57.0994, -55.8103) -> (-56.5994, -56.3103) centre (-56.5994, -55.8103) ccw
  line L223 (-55.3728, -54.5838) -> (-56.326, -54.5838)
  line L224 (-54.5994, -55.8103) -> (-54.5994, -54.3103)
  arc A111 (-55.0994, -56.3103) -> (-54.5994, -55.8103) centre (-55.0994, -55.8103) ccw
  line L225 (-55.3728, -55.5369) -> (-55.3728, -54.5838)
  line L226 (-56.326, -55.5369) -> (-55.3728, -55.5369)
  line L227 (-56.5994, -56.3103) -> (-55.0994, -56.3103)
  arc A112 (-52.0599, -54.3103) -> (-52.5599, -53.8103) centre (-52.5599, -54.3103) ccw
  line L228 (-52.5599, -53.8103) -> (-54.0599, -53.8103)
  line L229 (-54.5599, -54.3103) -> (-54.5599, -55.8103)
  arc A113 (-54.0599, -53.8103) -> (-54.5599, -54.3103) centre (-54.0599, -54.3103) ccw
  line L230 (-53.7865, -54.5838) -> (-53.7865, -55.5369)
  arc A114 (-54.5599, -55.8103) -> (-54.0599, -56.3103) centre (-54.0599, -55.8103) ccw
  line L231 (-52.8333, -54.5838) -> (-53.7865, -54.5838)
  line L232 (-52.0599, -55.8103) -> (-52.0599, -54.3103)
  arc A115 (-52.5599, -56.3103) -> (-52.0599, -55.8103) centre (-52.5599, -55.8103) ccw
  line L233 (-52.8333, -55.5369) -> (-52.8333, -54.5838)
  line L234 (-53.7865, -55.5369) -> (-52.8333, -55.5369)
  line L235 (-54.0599, -56.3103) -> (-52.5599, -56.3103)
  arc A116 (-49.5204, -54.3103) -> (-50.0204, -53.8103) centre (-50.0204, -54.3103) ccw
  line L236 (-50.0204, -53.8103) -> (-51.5204, -53.8103)
  line L237 (-52.0204, -54.3103) -> (-52.0204, -55.8103)
  arc A117 (-51.5204, -53.8103) -> (-52.0204, -54.3103) centre (-51.5204, -54.3103) ccw
  line L238 (-51.247, -54.5838) -> (-51.247, -55.5369)
  arc A118 (-52.0204, -55.8103) -> (-51.5204, -56.3103) centre (-51.5204, -55.8103) ccw
  line L239 (-50.2939, -54.5838) -> (-51.247, -54.5838)
  line L240 (-49.5204, -55.8103) -> (-49.5204, -54.3103)
  arc A119 (-50.0204, -56.3103) -> (-49.5204, -55.8103) centre (-50.0204, -55.8103) ccw
  line L241 (-50.2939, -55.5369) -> (-50.2939, -54.5838)
  line L242 (-51.247, -55.5369) -> (-50.2939, -55.5369)
  line L243 (-51.5204, -56.3103) -> (-50.0204, -56.3103)
  arc A120 (-46.981, -54.3103) -> (-47.481, -53.8103) centre (-47.481, -54.3103) ccw
  line L244 (-47.481, -53.8103) -> (-48.981, -53.8103)
  line L245 (-49.481, -54.3103) -> (-49.481, -55.8103)
  arc A121 (-48.981, -53.8103) -> (-49.481, -54.3103) centre (-48.981, -54.3103) ccw
  line L246 (-48.7076, -54.5838) -> (-48.7076, -55.5369)
  arc A122 (-49.481, -55.8103) -> (-48.981, -56.3103) centre (-48.981, -55.8103) ccw
  line L247 (-47.7544, -54.5838) -> (-48.7076, -54.5838)
  line L248 (-46.981, -55.8103) -> (-46.981, -54.3103)
  arc A123 (-47.481, -56.3103) -> (-46.981, -55.8103) centre (-47.481, -55.8103) ccw
  line L249 (-47.7544, -55.5369) -> (-47.7544, -54.5838)
  line L250 (-48.7076, -55.5369) -> (-47.7544, -55.5369)
  line L251 (-48.981, -56.3103) -> (-47.481, -56.3103)
  arc A124 (-44.4415, -54.3103) -> (-44.9415, -53.8103) centre (-44.9415, -54.3103) ccw
  line L252 (-44.9415, -53.8103) -> (-46.4415, -53.8103)
  line L253 (-46.9415, -54.3103) -> (-46.9415, -55.8103)
  arc A125 (-46.4415, -53.8103) -> (-46.9415, -54.3103) centre (-46.4415, -54.3103) ccw
  line L254 (-46.1681, -54.5838) -> (-46.1681, -55.5369)
  arc A126 (-46.9415, -55.8103) -> (-46.4415, -56.3103) centre (-46.4415, -55.8103) ccw
  line L255 (-45.2149, -54.5838) -> (-46.1681, -54.5838)
  line L256 (-44.4415, -55.8103) -> (-44.4415, -54.3103)
  arc A127 (-44.9415, -56.3103) -> (-44.4415, -55.8103) centre (-44.9415, -55.8103) ccw
  line L257 (-45.2149, -55.5369) -> (-45.2149, -54.5838)
  line L258 (-46.1681, -55.5369) -> (-45.2149, -55.5369)
  line L259 (-46.4415, -56.3103) -> (-44.9415, -56.3103)
  arc A128 (-41.902, -54.3103) -> (-42.402, -53.8103) centre (-42.402, -54.3103) ccw
  line L260 (-42.402, -53.8103) -> (-43.902, -53.8103)
  line L261 (-44.402, -54.3103) -> (-44.402, -55.8103)
  arc A129 (-43.902, -53.8103) -> (-44.402, -54.3103) centre (-43.902, -54.3103) ccw
  line L262 (-43.6286, -54.5838) -> (-43.6286, -55.5369)
  arc A130 (-44.402, -55.8103) -> (-43.902, -56.3103) centre (-43.902, -55.8103) ccw
  line L263 (-42.6755, -54.5838) -> (-43.6286, -54.5838)
  line L264 (-41.902, -55.8103) -> (-41.902, -54.3103)
  arc A131 (-42.402, -56.3103) -> (-41.902, -55.8103) centre (-42.402, -55.8103) ccw
  line L265 (-42.6755, -55.5369) -> (-42.6755, -54.5838)
  line L266 (-43.6286, -55.5369) -> (-42.6755, -55.5369)
  line L267 (-43.902, -56.3103) -> (-42.402, -56.3103)
  arc A132 (-39.3626, -54.3103) -> (-39.8626, -53.8103) centre (-39.8626, -54.3103) ccw
  line L268 (-39.8626, -53.8103) -> (-41.3626, -53.8103)
  line L269 (-41.8626, -54.3103) -> (-41.8626, -55.8103)
  arc A133 (-41.3626, -53.8103) -> (-41.8626, -54.3103) centre (-41.3626, -54.3103) ccw
  line L270 (-41.0891, -54.5838) -> (-41.0891, -55.5369)
  arc A134 (-41.8626, -55.8103) -> (-41.3626, -56.3103) centre (-41.3626, -55.8103) ccw
  line L271 (-40.136, -54.5838) -> (-41.0891, -54.5838)
  line L272 (-39.3626, -55.8103) -> (-39.3626, -54.3103)
  arc A135 (-39.8626, -56.3103) -> (-39.3626, -55.8103) centre (-39.8626, -55.8103) ccw
  line L273 (-40.136, -55.5369) -> (-40.136, -54.5838)
  line L274 (-41.0891, -55.5369) -> (-40.136, -55.5369)
  line L275 (-41.3626, -56.3103) -> (-39.8626, -56.3103)
  arc A136 (-36.8231, -54.3103) -> (-37.3231, -53.8103) centre (-37.3231, -54.3103) ccw
  line L276 (-37.3231, -53.8103) -> (-38.8231, -53.8103)
  line L277 (-39.3231, -54.3103) -> (-39.3231, -55.8103)
  arc A137 (-38.8231, -53.8103) -> (-39.3231, -54.3103) centre (-38.8231, -54.3103) ccw
  line L278 (-38.5497, -54.5838) -> (-38.5497, -55.5369)
  arc A138 (-39.3231, -55.8103) -> (-38.8231, -56.3103) centre (-38.8231, -55.8103) ccw
  line L279 (-37.5965, -54.5838) -> (-38.5497, -54.5838)
  line L280 (-36.8231, -55.8103) -> (-36.8231, -54.3103)
  arc A139 (-37.3231, -56.3103) -> (-36.8231, -55.8103) centre (-37.3231, -55.8103) ccw
  line L281 (-37.5965, -55.5369) -> (-37.5965, -54.5838)
  line L282 (-38.5497, -55.5369) -> (-37.5965, -55.5369)
  line L283 (-38.8231, -56.3103) -> (-37.3231, -56.3103)
  arc A140 (-34.2836, -54.3103) -> (-34.7836, -53.8103) centre (-34.7836, -54.3103) ccw
  line L284 (-34.7836, -53.8103) -> (-36.2836, -53.8103)
  line L285 (-36.7836, -54.3103) -> (-36.7836, -55.8103)
  arc A141 (-36.2836, -53.8103) -> (-36.7836, -54.3103) centre (-36.2836, -54.3103) ccw
  line L286 (-36.0102, -54.5838) -> (-36.0102, -55.5369)
  arc A142 (-36.7836, -55.8103) -> (-36.2836, -56.3103) centre (-36.2836, -55.8103) ccw
  line L287 (-35.057, -54.5838) -> (-36.0102, -54.5838)
  line L288 (-34.2836, -55.8103) -> (-34.2836, -54.3103)
  arc A143 (-34.7836, -56.3103) -> (-34.2836, -55.8103) centre (-34.7836, -55.8103) ccw
  line L289 (-35.057, -55.5369) -> (-35.057, -54.5838)
  line L290 (-36.0102, -55.5369) -> (-35.057, -55.5369)
  line L291 (-36.2836, -56.3103) -> (-34.7836, -56.3103)
  arc A144 (-31.7441, -54.3103) -> (-32.2441, -53.8103) centre (-32.2441, -54.3103) ccw
  line L292 (-32.2441, -53.8103) -> (-33.7441, -53.8103)
  line L293 (-34.2441, -54.3103) -> (-34.2441, -55.8103)
  arc A145 (-33.7441, -53.8103) -> (-34.2441, -54.3103) centre (-33.7441, -54.3103) ccw
  line L294 (-33.4707, -54.5838) -> (-33.4707, -55.5369)
  arc A146 (-34.2441, -55.8103) -> (-33.7441, -56.3103) centre (-33.7441, -55.8103) ccw
  line L295 (-32.5176, -54.5838) -> (-33.4707, -54.5838)
  line L296 (-31.7441, -55.8103) -> (-31.7441, -54.3103)
  arc A147 (-32.2441, -56.3103) -> (-31.7441, -55.8103) centre (-32.2441, -55.8103) ccw
  line L297 (-32.5176, -55.5369) -> (-32.5176, -54.5838)
  line L298 (-33.4707, -55.5369) -> (-32.5176, -55.5369)
  line L299 (-33.7441, -56.3103) -> (-32.2441, -56.3103)
  arc A148 (-29.2047, -54.3103) -> (-29.7047, -53.8103) centre (-29.7047, -54.3103) ccw
  line L300 (-29.7047, -53.8103) -> (-31.2047, -53.8103)
  line L301 (-31.7047, -54.3103) -> (-31.7047, -55.8103)
  arc A149 (-31.2047, -53.8103) -> (-31.7047, -54.3103) centre (-31.2047, -54.3103) ccw
  line L302 (-30.9312, -54.5838) -> (-30.9312, -55.5369)
  arc A150 (-31.7047, -55.8103) -> (-31.2047, -56.3103) centre (-31.2047, -55.8103) ccw
  line L303 (-29.9781, -54.5838) -> (-30.9312, -54.5838)
  line L304 (-29.2047, -55.8103) -> (-29.2047, -54.3103)
  arc A151 (-29.7047, -56.3103) -> (-29.2047, -55.8103) centre (-29.7047, -55.8103) ccw
  line L305 (-29.9781, -55.5369) -> (-29.9781, -54.5838)
  line L306 (-30.9312, -55.5369) -> (-29.9781, -55.5369)
  line L307 (-31.2047, -56.3103) -> (-29.7047, -56.3103)
  arc A152 (-26.6652, -54.3103) -> (-27.1652, -53.8103) centre (-27.1652, -54.3103) ccw
  line L308 (-27.1652, -53.8103) -> (-28.6652, -53.8103)
  line L309 (-29.1652, -54.3103) -> (-29.1652, -55.8103)
  arc A153 (-28.6652, -53.8103) -> (-29.1652, -54.3103) centre (-28.6652, -54.3103) ccw
  line L310 (-28.3918, -54.5838) -> (-28.3918, -55.5369)
  arc A154 (-29.1652, -55.8103) -> (-28.6652, -56.3103) centre (-28.6652, -55.8103) ccw
  line L311 (-27.4386, -54.5838) -> (-28.3918, -54.5838)
  line L312 (-26.6652, -55.8103) -> (-26.6652, -54.3103)
  arc A155 (-27.1652, -56.3103) -> (-26.6652, -55.8103) centre (-27.1652, -55.8103) ccw
  line L313 (-27.4386, -55.5369) -> (-27.4386, -54.5838)
  line L314 (-28.3918, -55.5369) -> (-27.4386, -55.5369)
  line L315 (-28.6652, -56.3103) -> (-27.1652, -56.3103)
  arc A156 (-24.1257, -54.3103) -> (-24.6257, -53.8103) centre (-24.6257, -54.3103) ccw
  line L316 (-24.6257, -53.8103) -> (-26.1257, -53.8103)
  line L317 (-26.6257, -54.3103) -> (-26.6257, -55.8103)
  arc A157 (-26.1257, -53.8103) -> (-26.6257, -54.3103) centre (-26.1257, -54.3103) ccw
  line L318 (-25.8523, -54.5838) -> (-25.8523, -55.5369)
  arc A158 (-26.6257, -55.8103) -> (-26.1257, -56.3103) centre (-26.1257, -55.8103) ccw
  line L319 (-24.8991, -54.5838) -> (-25.8523, -54.5838)
  line L320 (-24.1257, -55.8103) -> (-24.1257, -54.3103)
  arc A159 (-24.6257, -56.3103) -> (-24.1257, -55.8103) centre (-24.6257, -55.8103) ccw
  line L321 (-24.8991, -55.5369) -> (-24.8991, -54.5838)
  line L322 (-25.8523, -55.5369) -> (-24.8991, -55.5369)
  line L323 (-26.1257, -56.3103) -> (-24.6257, -56.3103)
  point P0 (-74.8757, -41.0103)
  point P1 (-72.3757, -41.0103)
  point P2 (-74.8757, -38.5103)
  point P3 (-72.3362, -38.5103)